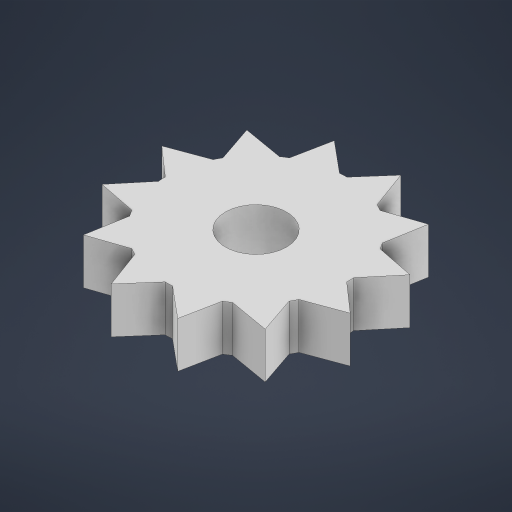
# Autodesk Inventor part: gir
Saved by Autodesk Inventor 2024.3 (Build 283343000, 343)
## iProperties
Created: 2025-06-30
Part Number: gir
Material: Generic
Document SubType Name: Modeling
Designer: Akbar Syihabuddin
Density: 1 g/cm^3
Appearance: Default
Author: Akbar Syihabuddin
Autodesk Inventor part; units mm, degrees
ref_plane "YZ Plane" through (0, 0, 0) normal (1, 0, 0) x (0, 1, 0)
ref_plane "XZ Plane" through (0, 0, 0) normal (0, 1, 0) x (-1, 0, 0)
ref_plane "XY Plane" through (0, 0, 0) normal (0, 0, 1) x (1, 0, 0)
sketch "Sketch1" plane through (0, 0, 0) normal (0, 1, 0) x (-1, 0, 0)
  circle A0 centre (0, 0) radius 2
  circle A1 centre (0, 0) radius 5.9473
  line L0 (5.3451, 5.9473) -> (2.9816, 5.146)
  line L1 (5.3451, 5.9473) -> (4.9023, 3.3673)
  line L2 (1.6553, 7.8231) -> (0.0091, 5.9473)
  line L3 (1.6553, 7.8231) -> (2.5618, 5.3673)
  line L4 (-2.478, 7.6027) -> (-2.9658, 5.1551)
  line L5 (-2.478, 7.6027) -> (-0.465, 5.9291)
  line L6 (-5.9473, 5.3451) -> (-5.146, 2.9816)
  line L7 (-5.9473, 5.3451) -> (-3.3673, 4.9023)
  line L8 (-7.8231, 1.6553) -> (-5.9473, 0.0091)
  line L9 (-7.8231, 1.6553) -> (-5.3673, 2.5618)
  line L10 (-7.6027, -2.478) -> (-5.1551, -2.9658)
  line L11 (-7.6027, -2.478) -> (-5.9291, -0.465)
  line L12 (-5.3451, -5.9473) -> (-2.9816, -5.146)
  line L13 (-5.3451, -5.9473) -> (-4.9023, -3.3673)
  line L14 (-1.6553, -7.8231) -> (-0.0091, -5.9473)
  line L15 (-1.6553, -7.8231) -> (-2.5618, -5.3673)
  line L16 (2.478, -7.6027) -> (2.9658, -5.1551)
  line L17 (2.478, -7.6027) -> (0.465, -5.9291)
  line L18 (5.9473, -5.3451) -> (5.146, -2.9816)
  line L19 (5.9473, -5.3451) -> (3.3673, -4.9023)
  line L20 (7.8231, -1.6553) -> (5.9473, -0.0091)
  line L21 (7.8231, -1.6553) -> (5.3673, -2.5618)
  line L22 (7.6027, 2.478) -> (5.1551, 2.9658)
  line L23 (7.6027, 2.478) -> (5.9291, 0.465)
  dimension "d0" = 4
  dimension "d3" = 360
  constraints: 48 end point, 2 coincident, 1 centre point, 65 other
  measures "d0" diameter of A0
extrude "Extrusion1" add sketch "Sketch1" along normal blind 3
body "Solid1"
